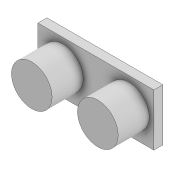
# Autodesk Inventor part: Sensor_Dummy
Saved by Autodesk Inventor 2020 (Build 240168000, 168)
## iProperties
Created: 2022-02-18
Part Number: Sensor_Dummy
Material: Generisch
Document SubType Name: Modeling
Designer: Julian Uhl
Density: 1 g/cm^3
Appearance: Vorgabe
Author: Julian Uhl
Autodesk Inventor part; units mm, degrees
ref_plane "YZ Plane" through (0, 0, 0) normal (1, 0, 0) x (0, 1, 0)
ref_plane "XZ Plane" through (0, 0, 0) normal (0, 1, 0) x (-1, 0, 0)
ref_plane "XY Plane" through (0, 0, 0) normal (0, 0, 1) x (1, 0, 0)
sketch "Skizze1" plane through (0, 0, 0) normal (0, 0, 1) x (1, 0, 0)
  line L0 (-9.02, 0) -> (54.12, 0) projected
  line L1 (0, -4.06) -> (0, 24.36) projected
  line L2 (0, 0) -> (45.1, 0)
  line L3 (45.1, 0) -> (45.1, 20.3)
  line L4 (45.1, 20.3) -> (0, 20.3)
  line L5 (0, 20.3) -> (0, 0)
  point P0 (0, 20.3)
  dimension "d0" = 20.3
  dimension "d1" = 45.1
  constraints: 8 end point, 2 parallel, 1 horizontal, 1 perpendicular
  measures "d0" distance between parallel lines of L0 L4
  measures "d1" distance between parallel lines of L3 L5
extrude "Extrusion1" add sketch "Skizze1" along normal blind 3.5
sketch "Skizze2" plane through (0, 0, 3.5) normal (0, 0, 1) x (1, 0, 0)
  circle A0 centre (35.4, 10.2) radius 7.9
  circle A1 centre (9.7, 10.2) radius 7.9
  line L0 (0, 20.3) -> (0, 0) projected
  line L1 (0, 0) -> (45.1, 0) projected
  dimension "d4" = 15.8
  dimension "d5" = 15.8
  dimension "d6" = 25.7
  dimension "d8" = 9.7
  dimension "d9" = 10.2
  dimension "d10" = 10.2
  constraints: 2 centre point
  measures "d4" diameter of A1
  measures "d5" diameter of A0
  measures "d6" distance of A0.centre A1.centre
  measures "d8" distance from line of L0 A1.centre
  measures "d9" distance from line of L1 A1.centre
  measures "d10" distance from line of L1 A0.centre
extrude "Extrusion2" add sketch "Skizze2" along normal blind 12.1
sketch "Skizze3" plane through (0, 0, 0) normal (0, 0, -1) x (-1, 0, 0)
  line L0 (-17.55, 2.7) -> (-27.55, 2.7)
  line L1 (-27.55, 2.7) -> (-27.55, 0.4)
  line L2 (-27.55, 0.4) -> (-17.55, 0.4)
  line L3 (-17.55, 0.4) -> (-17.55, 2.7)
  line L4 (0, 0) -> (-45.1, 0) projected
  line L5 (-45.1, 0) -> (-45.1, 20.3) projected
  dimension "d13" = 2.7
  dimension "d14" = 2.3
  dimension "d17" = 10
  dimension "d18" = 17.55
  constraints: 8 end point, 2 parallel, 1 horizontal, 1 perpendicular
  measures "d13" distance between parallel lines of L4 L0
  measures "d14" distance between parallel lines of L2 L0
  measures "d17" distance between parallel lines of L1 L3
  measures "d18" distance between parallel lines of L5 L1
extrude "Extrusion3" add sketch "Skizze3" along normal blind 4
